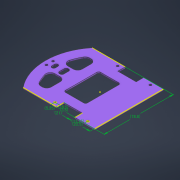
# Autodesk Inventor part: top
Saved by Autodesk Inventor 2022 (Build 260153000, 153)
## iProperties
Created: 2021-10-12
Part Number: top
Material: CFRP
Document SubType Name: Modeling
Designer: shiok
Density: 1.43 g/cm^3
Appearance: カーボンファイバー
Mass: 26.7457 g
Surface Area: 243.408 cm^2
Volume: 18.7033 cm^3
Author: shiok
Autodesk Inventor part; units mm, degrees
note: some values were not read from the file. Chosen so that the rebuilt part matches the saved one: direction of "穴2".
ref_plane "YZ Plane" through (0, 0, 0) normal (1, 0, 0) x (0, 1, 0)
ref_plane "XZ Plane" through (0, 0, 0) normal (0, 1, 0) x (-1, 0, 0)
ref_plane "XY Plane" through (0, 0, 0) normal (0, 0, 1) x (1, 0, 0)
sketch "スケッチ1" plane through (0, 0, 0) normal (0, 1, 0) x (-1, 0, 0)
  line L0 (62.5, 0) -> (-62.5, 0)
  line L1 (-10.5, -39.4) -> (-10.5, -30.9)
  line L2 (-10.5, -30.9) -> (10.5, -30.9)
  line L3 (10.5, -30.9) -> (10.5, -39.4)
  line L4 (0, -30.9) -> (0, -42.5)
  line L5 (0, 62.5) -> (0, -62.5)
  line L6 (-10.5, 39.4) -> (-10.5, 30.9)
  line L7 (-10.5, 30.9) -> (10.5, 30.9)
  line L8 (10.5, 30.9) -> (10.5, 39.4)
  line L9 (23, -39.4) -> (10.5, -39.4)
  line L10 (-10.5, -39.4) -> (-33, -39.4)
  line L11 (23, 58.1141) -> (23, 39.4)
  line L12 (23, -39.4) -> (23, -58.1141)
  line L13 (23, 39.4) -> (10.5, 39.4)
  arc A0 (23, -58.1141) -> (23, 58.1141) centre (0, 0) ccw
  arc A1 (23, 58.1141) -> (23, -58.1141) centre (0, 0) ccw construction
  line L14 (-33, 0) -> (-33, -39.4)
  line L15 (-10.5, 39.4) -> (-33, 39.4)
  line L16 (-33, 0) -> (-33, 39.4)
  line L17 (23, -39.4) -> (48.5169, -39.4)
  line L18 (23, 39.4) -> (48.5169, 39.4)
  point P0 (15.75, -35.9)
  point P1 (-21.75, -35.9)
  point P2 (15.75, 35.9)
  point P3 (-21.75, 35.9)
  point P4 (-23, -39.4)
  dimension "d1" = 37.5
  dimension "d2" = 21.75
  dimension "d4" = 35.9
  dimension "d8" = 21
  dimension "d27" = 23
  dimension "d30" = 62.5
  dimension "d50" = 22.5
  dimension "d73" = 78.8
  dimension "d74" = 8.5
  constraints: 38 end point, 10 point on circle, 8 symmetric about line, 4 midpoint, 3 horizontal, 3 point on line, 3 vertical, 2 centre point, 2 collinear, 1 coincident, 1 horizontal alignment, 1 parallel, 1 perpendicular
  measures "d1" distance of point (-21.75, -35.9) point (15.75, -35.9)
  measures "d2" horizontal distance of point (0, 0) point (-21.75, -35.9)
  measures "d4" vertical distance of point (0, 0) point (-21.75, -35.9)
  measures "d8" distance between parallel lines of L1 L3
  measures "d27" distance from line of L12 point (0, 0)
  measures "d30" radius of A0
  measures "d50" distance between parallel lines of L1 L14
  measures "d73" distance between parallel lines of L10 L15
  measures "d74" distance between parallel lines of L9 L2
extrude "押し出し1" add sketch "スケッチ1" along normal blind 1.6 contours A0 L17 L9 L3 L2 L5 L0 | L0 L5 L7 L8 L13 L18 A0 | L5 L2 L1 L10 L14 L0 | L0 L16 L15 L6 L7 L5
sketch "スケッチ2" plane through (0, 1.6, 0) normal (0, 1, 0) x (1, 0, 0)
  line L0 (62.5, 0) -> (-62.5, 0)
  point P0 (0, 0)
  point P1 (0, 0)
  point P2 (-15.75, 35.9)
  point P3 (21.75, 35.9)
  point P4 (0, 0)
  point P5 (21.75, -35.9)
  point P6 (-15.75, -35.9)
  dimension "d14" = 37.5
  dimension "d15" = 21.75
  dimension "d16" = 35.9
  constraints: 2 end point, 2 midpoint, 2 symmetric about line, 1 horizontal
  measures "d14" distance of point (21.75, 35.9) point (-15.75, 35.9)
  measures "d15" horizontal distance of point (0, 0) point (21.75, 35.9)
  measures "d16" vertical distance of point (0, 0) point (21.75, 35.9)
hole "穴1" at (21.75, 1.6, -35.9) at (-15.75, 1.6, -35.9) at (-15.75, 1.6, 35.9) at (21.75, 1.6, 35.9) direction (0, -1, 0) diameter 2.4 end through all clearance for "Countersunk Flat Head Screw ISO 2009/7046" size "M2" standard "ISO"
sketch "スケッチ3" plane through (0, 1.6, 0) normal (0, 1, 0) x (1, 0, 0)
  arc A0 (-48.5169, 39.4) -> (-48.5169, -39.4) centre (0, 0) ccw projected
  point P0 (-57.5, 3.75)
  point P1 (-57.5, -3.75)
  point P2 (-62.5, 0)
  point P3 (-23, 58.1141)
  point P4 (-23, -58.1141)
  point P5 (-47.1726, 41)
  dimension "d33" = 57.5
  dimension "d34" = 7.5
  dimension "d35" = 3.75
  constraints: 1 point on circle, 1 vertical alignment
  measures "d33" horizontal distance of point (0, 0) point (-57.5, -3.75)
  measures "d34" distance of point (-57.5, 3.75) point (-57.5, -3.75)
  measures "d35" vertical distance of point (0, 0) point (-57.5, -3.75)
hole "穴2" at (-57.5, 1.6, 3.75) at (-57.5, 1.6, -3.75) direction (0, -1, 0) diameter 2.4 depth 1.6 clearance for "Countersunk Flat Head Screw ISO 2009/7046" size "M2" standard "ISO"
sketch "スケッチ4" plane through (0, 1.6, 0) normal (0, 1, 0) x (1, 0, 0)
  line L0 (-19.5, 20) -> (1.5, 20)
  line L1 (3.5, 18) -> (3.5, -18)
  line L2 (1.5, -20) -> (-19.5, -20)
  line L3 (-21.5, -18) -> (-21.5, 18)
  line L4 (-22.6562, 0) -> (23.8715, 0)
  line L5 (-21.5, 20) -> (3.5, -20) construction
  line L6 (3.5, 20) -> (-21.5, -20) construction
  arc A0 (-19.5, 20) -> (-21.5, 18) centre (-19.5, 18) ccw
  arc A1 (3.5, 18) -> (1.5, 20) centre (1.5, 18) ccw
  arc A2 (1.5, -20) -> (3.5, -18) centre (1.5, -18) ccw
  arc A3 (-21.5, -18) -> (-19.5, -20) centre (-19.5, -18) ccw
  point P0 (-9, 0)
  point P1 (0, 0)
  dimension "d43" = 25
  dimension "d44" = 40
  dimension "d45" = 2
  dimension "d66" = 9
  constraints: 14 end point, 9 point on line, 8 point on circle, 8 tangent, 4 centre point, 3 equal radius, 2 horizontal, 2 parallel, 1 midpoint, 1 perpendicular, 1 other
  measures "d43" distance of L5.start L6.start
  measures "d44" distance of L6.start L5.end
  measures "d45" radius of A0
  measures "d66" distance of point (-9, 0) point (0, 0)
extrude "押し出し2" cut sketch "スケッチ4" against normal up to surface (1.6 mm away)
sketch "スケッチ5" plane through (0, 1.6, 0) normal (0, 1, 0) x (1, 0, 0)
  arc A0 (-44.2311, 25.3891) -> (-49.0809, 13.8587) centre (0, 0) ccw
  line L0 (-21.5, -18) -> (-21.5, 18) projected
  line L1 (-33, 22.9) -> (-33, 12.5)
  arc A1 (-48.5169, 39.4) -> (-48.5169, -39.4) centre (0, 0) ccw projected
  line L2 (-10.5, 39.4) -> (-48.5169, 39.4) construction
  arc A2 (-50.4474, 39.4) -> (-38.9474, 27.9) centre (-38.9474, 39.4) ccw construction
  line L3 (-51, 0) -> (-33, 0)
  line L4 (-39.8947, 27.9) -> (-38, 27.9)
  arc A3 (-49.0809, -13.8587) -> (-44.2311, -25.3891) centre (0, 0) ccw
  line L5 (-33, -22.9) -> (-33, -12.5)
  line L6 (-39.8947, -27.9) -> (-38, -27.9)
  line L7 (-44.2691, 7.5) -> (-38, 7.5)
  line L8 (-38, -7.5) -> (-44.2691, -7.5)
  arc A4 (-44.2691, -7.5) -> (-49.0809, -13.8587) centre (-44.2691, -12.5) ccw
  arc A5 (-49.0809, 13.8587) -> (-44.2691, 7.5) centre (-44.2691, 12.5) ccw
  arc A6 (-33, -12.5) -> (-38, -7.5) centre (-38, -12.5) ccw
  arc A7 (-38, -27.9) -> (-33, -22.9) centre (-38, -22.9) ccw
  arc A8 (-44.2311, -25.3891) -> (-39.8947, -27.9) centre (-39.8947, -22.9) ccw
  arc A9 (-38, 7.5) -> (-33, 12.5) centre (-38, 12.5) ccw
  arc A10 (-33, 22.9) -> (-38, 27.9) centre (-38, 22.9) ccw
  arc A11 (-39.8947, 27.9) -> (-44.2311, 25.3891) centre (-39.8947, 22.9) ccw
  line L9 (-41.6345, 5) -> (-40.6345, 5)
  line L10 (-38.6345, 3) -> (-38.6345, -3)
  line L11 (-40.6345, -5) -> (-41.6345, -5)
  line L12 (-43.6345, -3) -> (-43.6345, 3)
  line L13 (-44.2691, 12.5) -> (-38, 12.5) construction
  line L14 (-44.2691, -12.5) -> (-38, -12.5) construction
  line L15 (-41.1345, -12.5) -> (-41.1345, 12.5) construction
  arc A12 (-41.6345, 5) -> (-43.6345, 3) centre (-41.6345, 3) ccw
  arc A13 (-38.6345, 3) -> (-40.6345, 5) centre (-40.6345, 3) ccw
  arc A14 (-40.6345, -5) -> (-38.6345, -3) centre (-40.6345, -3) ccw
  arc A15 (-43.6345, -3) -> (-41.6345, -5) centre (-41.6345, -3) ccw
  line L16 (-33, 14.5) -> (-21.5, 14.5) construction
  line L17 (-10.5, 39.4) -> (-48.5169, 39.4) projected
  line L18 (-38.9474, 27.9) -> (-38.9474, 39.4) construction
  line L19 (-44.1673, 25.5) -> (-54.1266, 31.25) construction
  point P0 (-42.6918, 27.9)
  point P1 (-33, 27.9)
  point P2 (-42.6918, -27.9)
  point P3 (-33, -27.9)
  point P4 (-50.4455, 7.5)
  point P5 (-33, 7.5)
  point P6 (-33, -7.5)
  point P7 (-50.4455, -7.5)
  point P8 (-24, 7.5)
  point P9 (-38.6345, -5)
  point P10 (-38.6345, 5)
  point P11 (-43.6345, -5)
  point P12 (-47.1726, 41)
  point P13 (-23, 58.1141)
  point P14 (-23, -58.1141)
  point P15 (-23, 39.4)
  dimension "d51" = 11.5
  dimension "d58" = 15
  dimension "d59" = 5
  dimension "d60" = 2.5
  dimension "d61" = 5
  dimension "d63" = 2
  dimension "d64" = 7
  dimension "d65" = 30
  constraints: 39 point on circle, 34 end point, 25 tangent, 24 point on line, 15 centre point, 10 equal radius, 4 horizontal, 4 parallel, 3 midpoint, 2 equal length, 2 perpendicular, 2 symmetric about line, 1 coincident, 1 vertical, 7 other
  measures "d51" distance between parallel lines of L0 L1
  measures "d58" distance between parallel lines of L7 L8
  measures "d59" radius of A4
  measures "d60" distance between parallel lines of L8 L11
  measures "d61" distance between parallel lines of L10 L12
  measures "d63" radius of A12
  measures "d64" distance between parallel lines of L16 L7
  measures "d65" angle of L7 L19
extrude "押し出し3" cut sketch "スケッチ5" against normal blind 5
sketch "スケッチ6" plane through (0, 1.6, 0) normal (0, 1, 0) x (1, 0, 0)
  circle A0 centre (-57.5, 3.75) radius 1.2 projected
  line L0 (-57.5, 3.75) -> (-57.5, -3.75)
  circle A1 centre (-57.5, -3.75) radius 1.2 projected
  line L1 (-53.5, 3.5) -> (-49.5, 3.5)
  line L2 (-49.5, 3.5) -> (-49.5, -3.5)
  line L3 (-49.5, -3.5) -> (-53.5, -3.5)
  line L4 (-53.5, -3.5) -> (-53.5, 3.5)
  line L5 (-53.5, 3.5) -> (-49.5, -3.5) construction
  line L6 (-53.5, -3.5) -> (-49.5, 3.5) construction
  line L7 (-57.5, 0) -> (-51.5, 0) construction
  point P0 (0, 0)
  dimension "d67" = 7
  dimension "d68" = 4
  dimension "d69" = 6
  constraints: 16 end point, 2 midpoint, 2 parallel, 2 perpendicular, 1 coincident, 1 horizontal, 1 vertical
  measures "d67" distance of L3.end L1.start
  measures "d68" distance of L1.start L1.end
  measures "d69" distance of L7.start L7.end
extrude "押し出し4" cut sketch "スケッチ6" against normal blind 10 contours L1 L2 L3 L4
fillet "フィレット1" radius 2 4 edges at (-53.5, 0.8, -3.5) (-53.5, 0.8, 3.5) (-49.5, 0.8, 3.5) (-49.5, 0.8, -3.5)
sketch "スケッチ9" plane through (0, 1.6, 0) normal (0, 1, 0) x (1, 0, 0)
  line L0 (10.5, -30.9) -> (10.5, -39.4) projected
  line L1 (-10.5, -39.4) -> (-10.5, -30.9) projected
  line L2 (-10.5, 39.4) -> (-48.5169, 39.4) projected
  line L3 (-48.5169, -39.4) -> (-10.5, -39.4) projected
  line L4 (33, -39.4) -> (33, 39.4) projected
  circle A0 centre (-15.75, -35.9) radius 1.2 projected
  circle A1 centre (21.75, -35.9) radius 1.2 projected
  point P0 (0, 0)
  dimension "d76" = 21
  dimension "d77" = 78.8
  dimension "d78" = 22.5
  dimension "d79" = 5.25
  dimension "d80" = 8.5
  dimension "d81" = 11.25
  dimension "d82" = 3.5
  measures "d76" distance between parallel lines of L0 L1
  measures "d77" distance between parallel lines of L2 L3
  measures "d78" distance between parallel lines of L4 L0
  measures "d79" distance from line of A0.centre L1
  measures "d80" distance of L1.start L1.end
  measures "d81" distance from line of L0 A1.centre
  measures "d82" distance from line of L3 A0.centre
